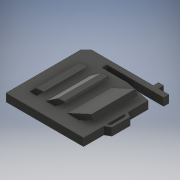
# Autodesk Inventor part: TA11
Saved by Autodesk Inventor 2017 (Build 210142000, 142)
## iProperties
Created: 2019-05-02
Part Number: TA11
Material: ABS Plastic
Document SubType Name: Modeling
Designer: Dell
Density: 1.06 g/cm^3
Appearance: Smooth - Black
Mass: 2.84891 g
Surface Area: 23.4524 cm^2
Volume: 2.68765 cm^3
Author: Dell
Autodesk Inventor part; units mm, degrees
ref_plane "YZ Plane" through (0, 0, 0) normal (1, 0, 0) x (0, 1, 0)
ref_plane "XZ Plane" through (0, 0, 0) normal (0, 1, 0) x (-1, 0, 0)
ref_plane "XY Plane" through (0, 0, 0) normal (0, 0, 1) x (1, 0, 0)
sketch "Sketch1" plane through (0, 0, 0) normal (0, 0, 1) x (1, 0, 0)
  line L0 (0, 0) -> (30, 0)
  line L1 (30, 0) -> (30, 27)
  line L2 (30, 27) -> (0, 27)
  line L3 (0, 27) -> (0, 0)
  dimension "d0" = 30
  dimension "d1" = 27
  constraints: 8 end point, 2 parallel, 1 horizontal, 1 perpendicular
  measures "d0" distance of L2.end L1.end
  measures "d1" distance of L1.end L0.end
extrude "Extrusion1" add sketch "Sketch1" along normal blind 3
sketch "Sketch2" plane through (0, 27, 0) normal (0, 1, 0) x (1, 0, 0)
  line L0 (0, 0) -> (0, -3) projected
  line L1 (0, 0) -> (30, 0) projected
  line L2 (0, -3) -> (10, -3)
  line L3 (10, -3) -> (10, 0)
  line L4 (10, 0) -> (0, 0)
  line L5 (0, 0) -> (0, -3)
  dimension "d4" = 10
  constraints: 8 end point, 2 parallel, 1 horizontal, 1 perpendicular, 1 point on line
  measures "d4" distance between parallel lines of L0 L3
extrude "Extrusion2" add sketch "Sketch2" along normal blind 2
sketch "Sketch3" plane through (0, 29, 0) normal (0, 1, 0) x (1, 0, 0)
  line L0 (0, 0) -> (0, -3) projected
  line L1 (0, -3) -> (32, -3)
  line L2 (32, -3) -> (32, 0)
  line L3 (32, 0) -> (0, 0)
  line L4 (0, 0) -> (0, -3)
  point P0 (30, 0)
  dimension "d7" = 2
  constraints: 8 end point, 2 parallel, 1 horizontal, 1 perpendicular, 1 point on line
  measures "d7" distance from line of point (30, 0) L2
extrude "Extrusion3" add sketch "Sketch3" along normal blind 2
chamfer "Chamfer1" distance 2 angle 45 1 edges at (0, 31, 1.5)
sketch "Sketch4" plane through (0, 0, 3) normal (0, 0, 1) x (1, 0, 0)
  line L0 (32, 29) -> (10, 29) projected
  line L1 (10, 29) -> (30, 24.9996)
  line L2 (10, 27) -> (10, 29) projected
  line L3 (30.3923, 26.9608) -> (10, 29)
  line L4 (10, 29) -> (10.3923, 30.9612) construction
  line L5 (10.3923, 30.9612) -> (30.3923, 26.9608) construction
  line L6 (30, 0) -> (30, 27) projected
  line L7 (30, 24.9996) -> (30.3923, 26.9608)
  point P0 (0, 0)
  dimension "d35" = 2
  dimension "d36" = 2
  constraints: 10 end point, 2 perpendicular, 2 point on line
  measures "d35" distance of L0.end L4.end
  measures "d36" distance of L3.start L1.end
extrude "Extrusion4" cut sketch "Sketch4" against normal through all contours L3 L6 L1
sketch "Sketch5" plane through (0, 0, 3) normal (0, 0, 1) x (1, 0, 0)
  line L0 (2, 31) -> (32, 31) projected
  line L1 (26, 31) -> (28, 31)
  line L2 (28, 31) -> (28, 33)
  line L3 (28, 33) -> (26, 33)
  line L4 (26, 33) -> (26, 31)
  line L5 (30, 0) -> (30, 24.9996) projected
  point P0 (0, 0)
  dimension "d16" = 2
  dimension "d17" = 2
  dimension "d18" = 2
  constraints: 8 end point, 2 parallel, 1 horizontal, 1 perpendicular, 1 point on line
  measures "d16" distance of L3.end L2.end
  measures "d17" distance of L3.end L1.start
  measures "d18" distance between parallel lines of L2 L5
extrude "Extrusion5" add sketch "Sketch5" against normal blind 3
sketch "Sketch6" plane through (0, 0, 3) normal (0, 0, 1) x (1, 0, 0)
  line L0 (30, 0) -> (30, 24.9996) projected
  line L1 (30, 17.1545) -> (32, 15.9998)
  line L2 (32, 15.9998) -> (32, 8.9998)
  line L3 (32, 8.9998) -> (30, 7.8451)
  line L4 (30, 8.9998) -> (31, 9.5772)
  line L5 (31, 9.5772) -> (31, 15.4225)
  line L6 (31, 15.4225) -> (30, 15.9998)
  line L7 (30, 7.8451) -> (30, 8.9998)
  line L8 (30, 17.1545) -> (30, 15.9998)
  point P0 (0, 0)
  point P1 (32, 12.4998)
  point P2 (30, 12.4998)
  dimension "d27" = 120
  dimension "d29" = 120
  dimension "d30" = 2
  dimension "d31" = 7
  dimension "d32" = 1
  constraints: 16 end point, 4 point on line, 2 midpoint, 1 horizontal alignment, 1 parallel, 2 other
  measures "d27" angle of L0 L1
  measures "d29" angle of L0 L3
  measures "d30" distance between parallel lines of L0 L2
  measures "d31" distance of L1.end L2.end
  measures "d32" distance between parallel lines of L2 L5
extrude "Extrusion6" add sketch "Sketch6" against normal blind 3 contours L0 L4 L5 L6 L1 L2 L3
ref_plane "Work Plane1" through (0, 5, 0) normal (0, -1, 0) x (1, 0, 0)
sketch "Sketch8" plane through (0, 5, 0) normal (0, -1, 0) x (1, 0, 0)
  line L0 (3.4995, 3) -> (4.4995, 6)
  line L1 (4.4995, 6) -> (6.4995, 6)
  line L2 (6.4995, 6) -> (7.4995, 3)
  line L3 (7.4995, 3) -> (8.4995, 6)
  line L4 (8.4995, 6) -> (11.4995, 6)
  line L5 (11.4995, 6) -> (12.4995, 3)
  line L6 (12.4995, 3) -> (13.4995, 6)
  line L7 (13.4995, 6) -> (16.4995, 6)
  line L8 (19.999, 3) -> (10, 3) construction
  line L9 (14.9995, 3) -> (14.9995, 6)
  line L10 (0, 3) -> (2, 3) construction
  line L11 (6.4995, 6) -> (8.4995, 6) construction
  line L12 (11.4995, 6) -> (13.4995, 6) construction
  line L13 (26.4995, 3) -> (25.4995, 6)
  line L14 (25.4995, 6) -> (23.4995, 6)
  line L15 (23.4995, 6) -> (22.4995, 3)
  line L16 (22.4995, 3) -> (21.4995, 6)
  line L17 (21.4995, 6) -> (18.4995, 6)
  line L18 (18.4995, 6) -> (17.4995, 3)
  line L19 (17.4995, 3) -> (16.4995, 6)
  line L20 (16.4995, 6) -> (13.4995, 6)
  line L21 (23.4995, 6) -> (21.4995, 6) construction
  line L22 (18.4995, 6) -> (16.4995, 6) construction
  line L23 (2.4454, 3) -> (3.7788, 7)
  line L24 (3.7788, 7) -> (7.2203, 7)
  line L25 (7.2203, 7) -> (7.4995, 6.1623)
  line L26 (7.4995, 6.1623) -> (7.7788, 7)
  line L27 (7.7788, 7) -> (12.2203, 7)
  line L28 (12.2203, 7) -> (12.4995, 6.1623)
  line L29 (12.4995, 6.1623) -> (12.7788, 7)
  line L30 (12.7788, 7) -> (16.4995, 7)
  line L31 (13.4995, 7) -> (17.2203, 7)
  line L32 (17.2203, 7) -> (17.4995, 6.1623)
  line L33 (17.4995, 6.1623) -> (17.7788, 7)
  line L34 (17.7788, 7) -> (22.2203, 7)
  line L35 (22.2203, 7) -> (22.4995, 6.1623)
  line L36 (22.4995, 6.1623) -> (22.7788, 7)
  line L37 (22.7788, 7) -> (26.2203, 7)
  line L38 (26.2203, 7) -> (27.5536, 3)
  line L39 (2, 3) -> (26, 3) construction
  line L40 (30, 3) -> (19.999, 3) construction
  line L41 (2.4454, 3) -> (3.4995, 3)
  line L42 (26.4995, 3) -> (27.5536, 3)
  line L43 (14.9995, 6) -> (14.9995, 7)
  line L44 (12.7788, 7) -> (14.9995, 7)
  line L45 (14.9995, 7) -> (17.2203, 7)
  line L46 (16.4995, 6) -> (14.9995, 6)
  line L47 (14.9995, 6) -> (13.4995, 6)
  line L48 (6.9995, 4.5) -> (7.9995, 4.5)
  line L49 (7.9995, 4.5) -> (7.9995, 3)
  line L50 (7.9995, 3) -> (6.9995, 3)
  line L51 (6.9995, 3) -> (6.9995, 4.5)
  line L52 (11.9995, 4.5) -> (12.9995, 4.5)
  line L53 (12.9995, 4.5) -> (12.9995, 3)
  line L54 (12.9995, 3) -> (11.9995, 3)
  line L55 (11.9995, 3) -> (11.9995, 4.5)
  line L56 (16.9995, 4.5) -> (17.9995, 4.5)
  line L57 (17.9995, 4.5) -> (17.9995, 3)
  line L58 (17.9995, 3) -> (16.9995, 3)
  line L59 (16.9995, 3) -> (16.9995, 4.5)
  line L60 (21.9995, 4.5) -> (22.9995, 4.5)
  line L61 (22.9995, 4.5) -> (22.9995, 3)
  line L62 (22.9995, 3) -> (21.9995, 3)
  line L63 (21.9995, 3) -> (21.9995, 4.5)
  line L64 (0, 3) -> (30, 3) construction
  line L65 (16.9995, 4.5) -> (17.9995, 4.5)
  line L66 (17.9995, 4.5) -> (17.9995, 3)
  line L67 (17.9995, 3) -> (16.9995, 3)
  line L68 (16.9995, 3) -> (16.9995, 4.5)
  line L69 (21.9995, 4.5) -> (22.9995, 4.5)
  line L70 (22.9995, 4.5) -> (22.9995, 3)
  line L71 (22.9995, 3) -> (21.9995, 3)
  line L72 (21.9995, 3) -> (21.9995, 4.5)
  point P0 (0, 0)
  point P1 (7.4995, 6)
  point P2 (12.4995, 6)
  point P3 (17.4995, 3)
  point P4 (22.4995, 3)
  dimension "d40" = 3
  dimension "d41" = 3
  dimension "d42" = 3
  dimension "d43" = 2
  dimension "d44" = 2
  dimension "d45" = 2
  dimension "d48" = 1
  dimension "d49" = 1
  dimension "d52" = 1
  dimension "d53" = 1
  dimension "d54" = 1
  constraints: 136 end point, 16 midpoint, 14 parallel, 9 collinear, 9 point on line, 9 symmetric about line, 8 perpendicular, 6 horizontal, 2 horizontal alignment, 2 vertical alignment, 14 other
  measures "d40" distance between parallel lines of L8 L1
  measures "d41" distance of L6.end L7.end
  measures "d42" distance of L3.end L4.end
  measures "d43" distance of L0.end L1.end
  measures "d44" distance of L6.end L4.end
  measures "d45" distance of L3.end L1.end
  measures "d48" distance between parallel lines of L0 L23
  measures "d49" distance between parallel lines of L19 L32
  measures "d52" distance between parallel lines of L61 L63
  measures "d53" distance of L52.start L52.end
  measures "d54" distance of L48.start L48.end
extrude "Extrusion7" [suppressed]
sketch "Sketch9" plane through (0, 5, 0) normal (0, -1, 0) x (1, 0, 0)
  line L0 (0, 3) -> (30, 3) projected
  line L1 (23.2369, 3) -> (29, 5.6874)
  line L2 (23.2369, 3) -> (29.5958, 3) construction
  line L3 (29, 5.6874) -> (28.1548, 7.5)
  line L4 (28.1548, 7.5) -> (18.5045, 3)
  line L5 (23.2369, 3) -> (18.5045, 3)
  line L6 (30, 0) -> (30, 3) projected
  line L7 (13.9131, 3) -> (18, 5.8617)
  line L8 (18, 5.8617) -> (16.8528, 7.5)
  line L9 (16.8528, 7.5) -> (10.4262, 3)
  line L10 (13.9131, 3) -> (10.4262, 3)
  line L11 (10.4262, 3) -> (13.9131, 3)
  line L12 (18.5045, 3) -> (23.2369, 3)
  line L13 (6.9142, 3) -> (10, 6.0858)
  line L14 (10, 6.0858) -> (8.5858, 7.5)
  line L15 (8.5858, 7.5) -> (4.0858, 3)
  line L16 (4.0858, 3) -> (6.9142, 3)
  point P0 (0, 0)
  dimension "d55" = 25
  dimension "d56" = 2
  dimension "d57" = 1
  dimension "d59" = 4.5
  dimension "d60" = 35
  dimension "d61" = 2
  dimension "d62" = 12
  dimension "d63" = 2
  dimension "d64" = 45
  dimension "d65" = 8
  constraints: 30 end point, 6 perpendicular, 6 point on line, 4 collinear, 2 horizontal, 2 horizontal alignment, 1 equal length
  measures "d55" angle of L2 L1
  measures "d56" distance of L1.end L3.end
  measures "d57" distance from line of L1.end L6
  measures "d59" vertical distance of L3.end L0.end
  measures "d60" angle of L0 L7
  measures "d61" distance of L7.end L8.end
  measures "d62" horizontal distance of L0.end L7.end
  measures "d63" distance of L13.end L14.end
  measures "d64" angle of L0 L13
  measures "d65" horizontal distance of L7.end L13.end
extrude "Extrusion8" add sketch "Sketch9" against normal blind 17
sketch "Sketch10" plane through (0, 5, 0) normal (0, -1, 0) x (1, 0, 0)
  line L0 (30, 7.6732) -> (-19.7811, 3)
  line L1 (-19.7811, 3) -> (-19.7811, 4.837)
  line L2 (-19.7811, 4.837) -> (29.8291, 9.4942)
  line L3 (29.8291, 9.4942) -> (30, 7.6732)
  point P0 (0, 0)
  point P1 (30, 3)
  point P2 (28.1548, 7.5)
  point P3 (0, 3)
  point P4 (8.5858, 7.5)
  dimension "d74" = 50
  constraints: 8 end point, 2 perpendicular, 2 point on line, 1 horizontal alignment, 1 vertical, 1 vertical alignment
  measures "d74" distance of L0.start L0.end
extrude "Extrusion9" cut sketch "Sketch10" against normal through all
body "Solid1"
